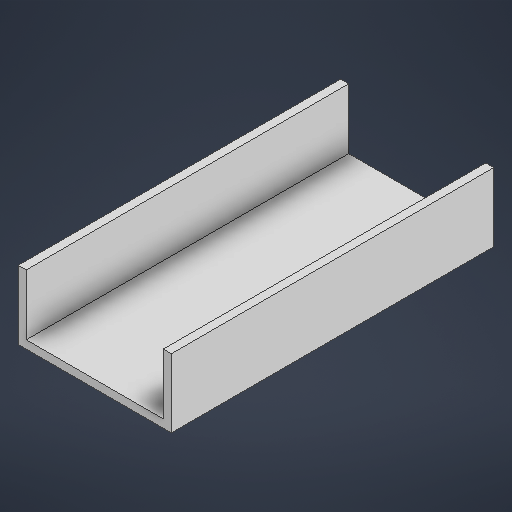
# Autodesk Inventor part: slide2
Saved by Autodesk Inventor 2026 (Build 300175000, 175)
## iProperties
Created: 2026-03-03
Part Number: slide2
Material: Generic
Document SubType Name: Modeling
Designer: shahd
Density: 1 g/cm^3
Appearance: Default
Author: shahd
Autodesk Inventor part; units mm, degrees
ref_plane "YZ Plane" through (0, 0, 0) normal (1, 0, 0) x (0, 1, 0)
ref_plane "XZ Plane" through (0, 0, 0) normal (0, 1, 0) x (-1, 0, 0)
ref_plane "XY Plane" through (0, 0, 0) normal (0, 0, 1) x (1, 0, 0)
sketch "Sketch1" plane through (0, 0, 0) normal (0, 0, 1) x (1, 0, 0)
  line L0 (2, 2) -> (36, 2)
  line L1 (36, 2) -> (36, 17)
  line L2 (2, 2) -> (2, 17)
  line L3 (0, 17) -> (0, 0)
  line L4 (0, 0) -> (38, 0)
  line L5 (38, 0) -> (38, 17)
  line L6 (0, 17) -> (2, 17)
  line L7 (36, 17) -> (38, 17)
  dimension "d0" = 34
  dimension "d1" = 15
  dimension "d2" = 15
  dimension "d3" = 2
  constraints: 16 end point, 3 horizontal, 2 perpendicular, 1 coincident, 1 vertical, 2 other
  measures "d0" distance of L0.start L0.end
  measures "d1" distance of L0.end L1.end
  measures "d2" distance of L0.start L2.end
  measures "d3" distance between parallel lines of L2 L3
extrude "Extrusion1" add sketch "Sketch1" along normal blind 80
body "Solid1"
